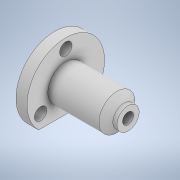
# Autodesk Inventor part: Деталь1
Saved by Autodesk Inventor 2022 (Build 260153000, 153)
## iProperties
Created: 2021-12-07
Part Number: Деталь1
Material: Типовые
Document SubType Name: Modeling
Designer: Украинцев
Density: 1 g/cm^3
Appearance: По умолчанию
Author: Украинцев
Autodesk Inventor part; units mm, degrees
ref_plane "YZ Plane" through (0, 0, 0) normal (1, 0, 0) x (0, 1, 0)
ref_plane "XZ Plane" through (0, 0, 0) normal (0, 1, 0) x (-1, 0, 0)
ref_plane "XY Plane" through (0, 0, 0) normal (0, 0, 1) x (1, 0, 0)
sketch "Эскиз1" plane through (0, 0, 0) normal (0, 1, 0) x (-1, 0, 0)
  line L0 (0, 9.5) -> (0, 14.5)
  line L1 (0, 14.5) -> (-2, 14.5)
  line L2 (-2, 14.5) -> (-2, 28)
  line L3 (-55, 4) -> (-55, 8)
  line L4 (-55, 8) -> (-52, 8)
  line L5 (-10, 28) -> (-10, 13)
  line L6 (-10, 13) -> (-47, 13)
  line L7 (-2, 14.5) -> (-2, 28)
  line L8 (-2, 28) -> (-10, 28)
  line L9 (-52, 8) -> (-47.3096, 12.6904)
  line L10 (-47.3096, 12.6904) -> (-47, 13)
  line L11 (0, 0) -> (0, 9.5)
  line L12 (0, 9.5) -> (-2, 9.5)
  line L13 (-2, 7.5) -> (-2, 9.5)
  line L14 (-2, 7.5) -> (-5.5, 7.5)
  line L15 (-5.5, 7.5) -> (-5.5, 9)
  line L16 (-5.5, 9) -> (-8, 9)
  line L17 (0, 0) -> (0, 7)
  line L18 (-8, 9) -> (-8, 0)
  line L19 (-30, 0) -> (-30, 8)
  line L20 (-30, 8) -> (-42, 8)
  line L21 (-42, 8) -> (-42, 6)
  line L22 (-55, 4) -> (-44, 4)
  line L23 (-42, 6) -> (-44, 4)
  line L24 (0, 0) -> (-55, 0)
  line L25 (-8, 0) -> (-30, 0)
  point P0 (-42, 4)
  dimension "d26" = 30
  dimension "d27" = 12
  dimension "d28" = 2
  dimension "d29" = 2
  dimension "d30" = 55
  dimension "d31" = 8
  dimension "d32" = 16
  dimension "d33" = 26
  dimension "d34" = 16
  dimension "d35" = 12
  dimension "d36" = 42
  dimension "d37" = 18
  dimension "d38" = 8
  dimension "d39" = 2.5
  dimension "d40" = 29
  dimension "d41" = 19
  dimension "d42" = 15
  dimension "d43" = 2
  dimension "d44" = 55
  dimension "d45" = 3
  dimension "d46" = 135
  dimension "d47" = 45
  dimension "d48" = 56
  dimension "d49" = 2
  constraints: 52 end point, 6 perpendicular, 5 vertical, 3 horizontal, 3 point on line, 1 collinear
  measures "d26" distance of L11.start L19.start
  measures "d27" distance of L19.end L20.end
  measures "d28" distance of L21.end point (-42, 4)
  measures "d29" distance of L22.end point (-42, 4)
  measures "d30" distance of L11.start L24.end
  measures "d31" diameter of L22 L24
  measures "d32" diameter of L4 L24
  measures "d33" diameter of L6 L24
  measures "d34" diameter of L20 L24
  measures "d35" distance between parallel lines of L19 L21
  measures "d36" distance between parallel lines of L0 L21
  measures "d37" diameter of L16 L24
  measures "d38" distance between parallel lines of L0 L18
  measures "d39" distance between parallel lines of L15 L18
  measures "d40" diameter of L1 L24
  measures "d41" diameter of L12 L24
  measures "d42" diameter of L14 L24
  measures "d43" distance between parallel lines of L0 L2
  measures "d44" distance between parallel lines of L3 L0
  measures "d45" distance of L3.end L4.end
  measures "d46" angle of L9 L4
  measures "d47" distance between parallel lines of L5 L3
  measures "d48" diameter of L8 L24
  measures "d49" distance between parallel lines of L11 L13
revolve "Вращение1" add sketch "Эскиз1" angle 360 about axis through (0, 0, 0) along (1, 0, 0) contours L12 L13 L14 L15 L16 L18 L24 L19 L20 L21 L23 L22 L3 L4 L9 L10 L6 L5 L8 L2 L1 L0
sketch "Эскиз3" plane through (8, 0, 0) normal (-1, 0, 0) x (0, 0, 1)
  point P0 (0, 0)
  point P1 (0, 0)
  constraints: 1 coincident
hole "Отверстие2" at (8, 0, 0) direction (1, 0, 0) diameter 12.376 depth 30 thread size "M14x1.5" class "6H" standard "ISO Metric profile"
sketch "Эскиз4" plane through (2, 0, 0) normal (-1, 0, 0) x (0, 0, 1)
  circle A0 centre (0, 0) radius 21
  point P0 (0, 21)
  dimension "d65" = 42
  constraints: 1 coincident, 1 vertical alignment, 2 other
chamfer "Фаска1" distance 2 angle 45 1 edges at (8, 0, -6.188)
sketch "Эскиз5" plane through (2, 0, 0) normal (-1, 0, 0) x (0, 0, 1)
  point P0 (0, 0)
hole "Отверстие4" at (2, 21, 0) direction (1, 0, 0) diameter 9 depth 30
pattern_circular "Круговой массив2" count 3 over 360 about axis through (1, 0, 0) along (-1, 0, 0) of "Отверстие4"
sketch "Эскиз6" plane through (2, 0, 0) normal (-1, 0, 0) x (0, 0, 1)
  circle A0 centre (0, 0) radius 28 projected
  line L0 (55.1219, -20) -> (-57.0995, -20)
  line L1 (55.1219, -20) -> (-57.0995, -20)
  line L2 (-57.0995, -20) -> (-57.0995, -35.8887)
  line L3 (-57.0995, -35.8887) -> (55.1219, -35.8887)
  line L4 (55.1219, -35.8887) -> (55.1219, -20)
  point P0 (0, 28)
  point P1 (19.5959, -20)
  point P2 (-19.5959, -20)
  dimension "d91" = 48
  constraints: 10 end point, 2 horizontal, 2 parallel, 1 perpendicular, 2 other
  measures "d91" distance from line of L0 point (0, 28)
extrude "Выдавливание1" cut sketch "Эскиз6" against normal blind 10 contours L0 A0 picked at (4.9079, -21.2721)
equation "\"d29\" = d28"
